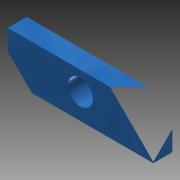
# Autodesk Inventor part: ZAxisNutMount
Saved by Autodesk Inventor 2015 SP1 (Build 190203100, 203)
## iProperties
Created: 2014-12-11
Part Number: ZAxisNutMount
Material: Generic
Document SubType Name: Modeling
Designer: Jack
Density: 1 g/cm^3
Appearance: Cyan
Author: Jack
Autodesk Inventor part; units mm, degrees
ref_plane "YZ Plane" through (0, 0, 0) normal (1, 0, 0) x (0, 1, 0)
ref_plane "XZ Plane" through (0, 0, 0) normal (0, 1, 0) x (-1, 0, 0)
ref_plane "XY Plane" through (0, 0, 0) normal (0, 0, 1) x (1, 0, 0)
sketch "Sketch1" plane through (0, 0, 0) normal (0, 0, 1) x (1, 0, 0)
  line L0 (0, 0) -> (92, 0)
  line L1 (92, 0) -> (92, 12)
  line L2 (92, 12) -> (0, 12)
  line L3 (0, 12) -> (0, 0)
  dimension "d0" = 92
  dimension "d1" = 12
  constraints: 8 end point, 2 parallel, 1 horizontal, 1 perpendicular
  measures "d0" distance of L2.end L1.end
  measures "d1" distance of L2.end L0.start
extrude "Extrusion1" add sketch "Sketch1" along normal blind 30
sketch "Sketch3" plane through (0, 12, 30) normal (0, 1, 0) x (1, 0, 0)
  line L0 (0, 30) -> (0, 0) projected
  line L1 (92, 30) -> (0, 30) projected
  circle A0 centre (46, 14.15) radius 7.9
  point P0 (0, 17)
  point P1 (107, 32)
  point P2 (15, 32)
  dimension "d8" = 15.8
  dimension "d9" = 15.85
  dimension "d10" = 46
  constraints: 1 centre point, 1 other
  measures "d8" diameter of A0
  measures "d10" distance from line of L0 A0.centre
extrude "Extrusion3" cut sketch "Sketch3" against normal up to next
sketch "Sketch4" plane through (0, 12, 0) normal (0, 1, 0) x (1, 0, 0)
  line L0 (0, 0) -> (0, -30) projected
  line L1 (92, 0) -> (92, -30) projected
  line L2 (0, -30) -> (-15, -15)
  line L3 (-15, -15) -> (0, -15)
  line L4 (92, -30) -> (107, -15)
  line L5 (107, -15) -> (92, -15)
  dimension "d13" = 45
  dimension "d14" = 45
  constraints: 8 end point, 2 midpoint, 1 perpendicular, 1 point on line
  measures "d13" angle of L1 L4
  measures "d14" angle of L0 L2
extrude "Extrusion4" add sketch "Sketch4" against normal up to surface (12 mm away)
body "Solid1"
